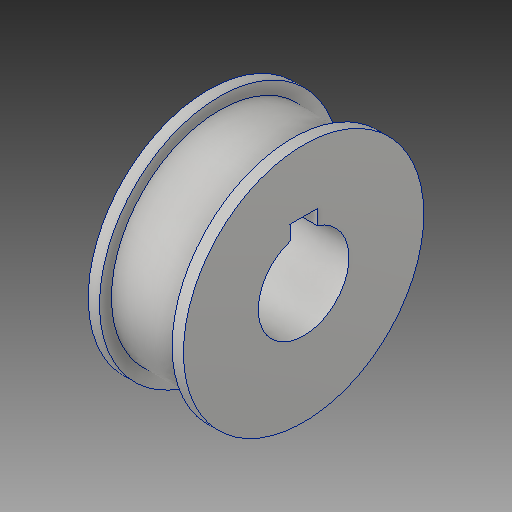
# Autodesk Inventor part: HTD 5M 30 20mm ID Keyed
Saved by Autodesk Inventor 2019.4 (Build 234330000, 330)
## iProperties
Created: 2020-01-05
Part Number: HTD 5M 30 20mm ID Keyed
Material: Aluminum 6061
Document SubType Name: Modeling
Designer: Mark
Mass: 88.327 g
Surface Area: 92.6662 cm^2
Volume: 32.7137 cm^3
Density: 2.7 g/cm^3
Appearance: Aluminum - Flat
Author: Mark
Autodesk Inventor part; units mm, degrees
ref_plane "YZ Plane" through (0, 0, 0) normal (1, 0, 0) x (0, 1, 0)
ref_plane "XZ Plane" through (0, 0, 0) normal (0, 1, 0) x (-1, 0, 0)
ref_plane "XY Plane" through (0, 0, 0) normal (0, 0, 1) x (1, 0, 0)
sketch "Sketch1" plane through (0, 0, 0) normal (1, 0, 0) x (0, 1, 0)
  circle A0 centre (65.4829, 84.7217) radius 26.5
  point P0 (0, 0)
  dimension "d0" = 53
  constraints: 1 centre point
  measures "d0" diameter of A0
extrude "Extrusion1" add sketch "Sketch1" along normal blind 2.5
sketch "Sketch2" plane through (2.5, 65.4829, 84.7217) normal (1, 0, 0) x (0, 0, -1)
  circle A0 centre (0, 0) radius 23.875
  circle A1 centre (0, 0) radius 26.5 projected
  point P0 (84.7217, -65.4829)
  dimension "d3" = 47.75
  constraints: 1 centre point, 1 concentric
  measures "d3" diameter of A0
extrude "Extrusion2" add sketch "Sketch2" along normal blind 16 contours A0
sketch "Sketch3" plane through (18.5, 65.4829, 84.7217) normal (1, 0, 0) x (0, 0, -1)
  circle A0 centre (0, 0) radius 26.5
  circle A1 centre (0, 0) radius 26.5 projected
  point P0 (84.7217, -65.4829)
  dimension "d6" = 53
  constraints: 1 centre point, 1 concentric
  measures "d6" diameter of A0
extrude "Extrusion3" add sketch "Sketch3" along normal blind 2.5
sketch "Sketch4" plane through (21, 65.4829, 84.7217) normal (1, 0, 0) x (0, 0, -1)
  circle A0 centre (0, 0) radius 10
  circle A1 centre (0, 0) radius 26.5 projected
  line L0 (-3, 12.8) -> (3, 12.8)
  line L1 (3, 12.8) -> (3, 7.2)
  line L2 (3, 7.2) -> (-3, 7.2)
  line L3 (-3, 7.2) -> (-3, 12.8)
  line L4 (-3, 12.8) -> (3, 7.2) construction
  line L5 (3, 12.8) -> (-3, 7.2) construction
  point P0 (84.7217, -65.4829)
  point P1 (0, 10)
  dimension "d9" = 20
  dimension "d10" = 6
  dimension "d11" = 5.6
  constraints: 12 end point, 2 midpoint, 2 parallel, 1 horizontal, 1 perpendicular, 1 vertical alignment, 3 other
  measures "d10" distance of L1.end L2.end
  measures "d11" distance of L0.end L1.end
extrude "Extrusion4" cut sketch "Sketch4" against normal blind 21 contours A0 L3 L2 L1 | L1 L2 L3 A0 | A0 L3 L0 L1
body "Solid1"
